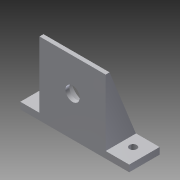
# Autodesk Inventor part: z leadscrew top mount
Saved by Autodesk Inventor 2014 SP1 (Build 180222100, 222)
## iProperties
Created: 2014-10-09
Part Number: z leadscrew top mount
Material: ABS Plastic
Document SubType Name: Modeling
Designer: Mon
Density: 1.06 g/cm^3
Appearance: Smooth - White
Author: Mon
Autodesk Inventor part; units mm, degrees
ref_plane "YZ Plane" through (0, 0, 0) normal (1, 0, 0) x (0, 1, 0)
ref_plane "XZ Plane" through (0, 0, 0) normal (0, 1, 0) x (-1, 0, 0)
ref_plane "XY Plane" through (0, 0, 0) normal (0, 0, 1) x (1, 0, 0)
sketch "Sketch6" plane through (0, 0, 0) normal (0, 0, 1) x (1, 0, 0)
  line L0 (0, 0) -> (82.3, 0)
  line L1 (82.3, 0) -> (82.3, 20)
  line L2 (82.3, 20) -> (0, 20)
  line L3 (0, 20) -> (0, 0)
  line L4 (0, 0) -> (10, 0) construction
  line L5 (10, 0) -> (10, 26.8607) construction
  line L6 (0, 10) -> (82.8633, 10) construction
  line L7 (82.3, 0) -> (72.3, 0) construction
  line L8 (72.3, 0) -> (72.3, 17.2228) construction
  circle A0 centre (10, 10) radius 2.75
  circle A1 centre (72.3, 10) radius 2.75
  dimension "d32" = 82.3
  dimension "d33" = 20
  dimension "d34" = 10
  dimension "d35" = 10
  dimension "d36" = 5.5
  dimension "d37" = 5.5
  constraints: 18 end point, 6 point on line, 4 perpendicular, 2 centre point, 2 parallel, 1 horizontal, 1 midpoint
  measures "d32" distance of L2.end L1.end
  measures "d33" distance of L1.end L0.end
  measures "d34" distance of L0.start L4.end
  measures "d35" distance of L0.end L7.end
  measures "d36" diameter of A0
  measures "d37" diameter of A1
extrude "Extrusion5" add sketch "Sketch6" along normal blind 5
sketch "Sketch7" plane through (0, 0, 0) normal (0, -1, 0) x (1, 0, 0)
  line L0 (82.3, 0) -> (82.3, 5) projected
  line L1 (0, 0) -> (0, 5) projected
  line L2 (41.15, 21.713) -> (41.15, -8.4757)
  line L3 (64.494, 5) -> (64.494, 55)
  line L4 (64.494, 55) -> (14.494, 55)
  line L5 (14.494, 55) -> (14.494, 5)
  line L6 (14.494, 5) -> (0, 5)
  line L7 (64.494, 5) -> (82.3, 5)
  line L8 (82.3, 0) -> (0, 0)
  dimension "d40" = 50
  dimension "d41" = 50
  constraints: 14 end point, 2 parallel, 1 perpendicular
  measures "d40" distance of L3.start L3.end
  measures "d41" distance of L3.end L4.end
extrude "Extrusion6" add sketch "Sketch7" along normal blind 3
sketch "Sketch8" plane through (64.494, 0, 55) normal (1, 0, 0) x (0, 0, -1)
  line L0 (0, 0) -> (50, 0) projected
  line L1 (0, 0) -> (50, 19.8426)
  line L2 (0, 0) -> (50, 0)
  line L3 (50, 0) -> (50, 19.8426)
  point P0 (55, 0)
  constraints: 6 end point, 1 collinear, 1 perpendicular
extrude "Extrusion7" add sketch "Sketch8" against normal blind 3
sketch "Sketch9" plane through (14.494, 0, 5) normal (-1, 0, 0) x (0, 0, 1)
  line L0 (50, 0) -> (50, -3) projected
  line L1 (0, 0) -> (50, 0)
  line L2 (50, 0) -> (0, 20.0433)
  line L3 (0, 0) -> (0, 20.0433)
  constraints: 6 end point, 2 perpendicular
extrude "Extrusion8" add sketch "Sketch9" against normal blind 3
sketch "Sketch10" plane through (0, 0, 0) normal (0, 1, 0) x (1, 0, 0)
  line L0 (17.494, -5) -> (61.494, -55) construction
  line L1 (61.494, -5) -> (17.494, -55) construction
  circle A0 centre (39.494, -30) radius 11.25
  circle A1 centre (39.494, -30) radius 12.25
  point P0 (0, 0)
  dimension "d48" = 22.5
  dimension "d49" = 24.5
  constraints: 4 end point, 3 midpoint, 2 centre point
  measures "d48" diameter of A0
  measures "d49" diameter of A1
extrude "Extrusion9" add sketch "Sketch10" along normal blind 7
sketch "Sketch11" plane through (39.494, 0, 30) normal (0, 1, 0) x (1, 0, 0)
  circle A0 centre (0, 0) radius 11.25 projected
  circle A1 centre (0, 0) radius 5.4
  point P0 (-39.494, 30)
  dimension "d52" = 10.8
  constraints: 1 centre point, 1 coincident
  measures "d52" diameter of A1
extrude "Extrusion10" cut sketch "Sketch11" against normal through all contours A1
body "Solid2"
